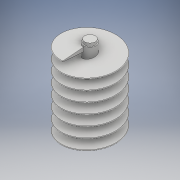
# Autodesk Inventor part: Infinite_screw
Saved by Autodesk Inventor 2018 (Build 220112000, 112)
## iProperties
Created: 2021-04-16
Part Number: Infinite_screw
Material: Generic
Document SubType Name: Modeling
Designer: danielcastro
Density: 1 g/cm^3
Appearance: Default
Author: danielcastro
Autodesk Inventor part; units mm, degrees
ref_plane "YZ Plane" through (0, 0, 0) normal (1, 0, 0) x (0, 1, 0)
ref_plane "XZ Plane" through (0, 0, 0) normal (0, 1, 0) x (-1, 0, 0)
ref_plane "XY Plane" through (0, 0, 0) normal (0, 0, 1) x (1, 0, 0)
sketch "Sketch1" plane through (0, 0, 0) normal (1, 0, 0) x (0, 1, 0)
  line L0 (0, 107) -> (0, -107)
  line L1 (0, -107) -> (12.7, -107)
  line L2 (12.7, -107) -> (12.7, -100)
  line L3 (12.7, -100) -> (15, -100)
  line L4 (15, -100) -> (15, 100)
  line L5 (15, 100) -> (12.7, 100)
  line L6 (12.7, 100) -> (12.7, 107)
  line L7 (12.7, 107) -> (0, 107)
  line L8 (0, 0) -> (15, 0) construction
  dimension "d1" = 25.4
  dimension "d2" = 7
  dimension "d3" = 7
  dimension "d4" = 200
  dimension "d5" = 30
  constraints: 18 end point, 6 perpendicular, 2 midpoint, 2 point on line, 1 horizontal, 1 vertical, 1 other
  measures "d1" diameter of L2 L0
  measures "d2" distance of L1.end L2.end
  measures "d3" distance of L5.end L6.end
  measures "d4" distance of L3.end L4.end
  measures "d5" diameter of L4 L0
revolve "Revolution1" add sketch "Sketch1" angle 360 about axis through (0, 0, 107) along (0, 0, -1)
sketch "Sketch2" plane through (0, 0, 0) normal (1, 0, 0) x (0, 1, 0)
  line L0 (-12.7, 107) -> (12.7, 107) projected
  line L1 (12.7, 107) -> (12.7, 100) projected
  line L2 (12.7, 100) -> (15, 100) projected
  line L3 (15, 100) -> (15, -100) projected
  line L4 (15, -100) -> (12.7, -100) projected
  line L5 (12.7, -100) -> (12.7, -107) projected
  line L6 (12.7, -107) -> (-12.7, -107) projected
  line L7 (-12.7, -107) -> (-12.7, -100) projected
  line L8 (-12.7, -100) -> (-15, -100) projected
  line L9 (-15, -100) -> (-15, 100) projected
  line L10 (-15, 100) -> (-12.7, 100) projected
  line L11 (-12.7, 100) -> (-12.7, 107) projected
  line L12 (15, -100) -> (65.8784, -95.9969)
  line L13 (65.8784, -94.0031) -> (15, -90)
  line L14 (78.5491, -95) -> (15, -95) construction
  line L15 (15, 100) -> (15, -100) projected
  arc A0 (65.8784, -95.9969) -> (65.8784, -94.0031) centre (65.8, -95) ccw
  line L16 (-12.7, 107) -> (12.7, 107) projected
  line L17 (0, 107) -> (0, -107)
  line L18 (-12.7, -107) -> (12.7, -107) projected
  line L19 (15, -90) -> (7.512, -90)
  line L20 (7.512, -90) -> (7.512, -100)
  line L21 (-15, -100) -> (15, -100) projected
  line L22 (7.512, -100) -> (15, -100)
  point P0 (0, 0)
  dimension "d8" = 10
  dimension "d9" = 1
  dimension "d10" = 50.8
  dimension "d11" = 7.488
  constraints: 14 end point, 4 point on line, 3 perpendicular, 2 midpoint, 2 point on circle, 2 tangent, 1 centre point, 1 horizontal, 1 other
  measures "d8" distance of L13.end L3.end
  measures "d9" radius of A0
  measures "d10" distance of L14.end A0.centre
  measures "d11" distance of L13.end L19.end
coil "Coil1" sketch "Sketch2" operation add axis through (0, 0, 107) along (0, 0, 1) pitch 25 turns 7.5 hand right contours L13 A0 L12 L3
equation "\"d3\" = d2"
body "Solid1"
